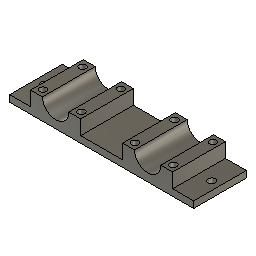
solenoid_railmount v2 (Autodesk Fusion 360 design; units mm, degrees)
Autodesk Fusion 360 part; units mm, degrees
note: some values were not read from the file. Set by a fixed rule: the direction of a hole.
sketch "Sketch1" plane through (0, 0, 0) normal (0, 0, 1) x (1, 0, 0)
  line L0 (0, 0) -> (139.7, 0)
  line L1 (139.7, 0) -> (139.7, 40)
  line L2 (139.7, 40) -> (0, 40)
  line L3 (0, 40) -> (0, 0)
  dimension "d1" = 139.7
  dimension "d2" = 40
  constraint horizontal L0
  constraint vertical L1
  constraint horizontal L2
  constraint vertical L3
  constraint coincident L0.start L3.end
  measures "d1" distance of L0.start L0.end
  measures "d2" distance of L0.start L2.end
extrude "Extrude1" add sketch "Sketch1" along normal blind 5
sketch "Sketch2" plane through (0, 0, 0) normal (0, 0, 1) x (1, 0, 0)
  point P0 (6.35, 20)
  point P1 (133.35, 20)
  constraint horizontal P0 P1
hole "Hole1" at (6.35, 20, 0) at (133.35, 20, 0) direction (0, 0, 1) diameter 5.5 depth 13 tip angle 118 counterbore diameter 9.1 counterbore depth 1
sketch "Sketch7" plane through (0, 0, 5) normal (0, 0, 1) x (-1, 0, 0)
  circle A0 centre (-6.35, -20) radius 2.75
  circle A1 centre (-133.35, -20) radius 2.75
  line L0 (0, -40) -> (0, 0)
  line L1 (0, 0) -> (-139.7, 0)
  line L2 (-139.7, 0) -> (-139.7, -40)
  line L3 (-139.7, -40) -> (0, -40)
  line L4 (-85.775, -40) -> (-123.775, -40)
  line L5 (-123.775, -40) -> (-123.775, 0)
  line L6 (-123.775, 0) -> (-85.775, 0)
  line L7 (-85.775, 0) -> (-85.775, -40)
  line L8 (-85.775, -40) -> (-123.775, 0) construction
  line L9 (-123.775, -40) -> (-85.775, 0) construction
  line L10 (-15.925, -40) -> (-53.925, -40)
  line L11 (-53.925, -40) -> (-53.925, 0)
  line L12 (-53.925, 0) -> (-15.925, 0)
  line L13 (-15.925, 0) -> (-15.925, -40)
  line L14 (-15.925, -40) -> (-53.925, 0) construction
  line L15 (-53.925, -40) -> (-15.925, 0) construction
  point P0 (-104.775, -20)
  point P1 (-34.925, -20)
  point P2 (-104.775, -20)
  point P3 (-34.925, -20)
  dimension "d25" = 38
  dimension "d26" = 40
  dimension "d27" = 38
  dimension "d28" = 40
  constraint horizontal L4
  constraint perpendicular L4 L5
  constraint parallel L4 L6
  constraint parallel L5 L7
  constraint coincident L8 P2
  constraint coincident L9 P2
  constraint coincident P2 P0
  constraint horizontal L10
  constraint perpendicular L10 L11
  constraint parallel L10 L12
  constraint parallel L11 L13
  constraint coincident L14 P3
  constraint coincident L15 P3
  constraint coincident P3 P1
  measures "d25" distance of L5.end L6.end
  measures "d26" distance of L4.end L5.end
  measures "d27" distance of L11.end L12.end
  measures "d28" distance of L10.end L11.end
extrude "Extrude4" add sketch "Sketch7" along normal blind 11 contours L1 L3 L10 L11 L12 L13 | L1 L3 L4 L5 L6 L7
sketch "Sketch8" plane through (0, 40, 0) normal (0, 1, 0) x (-1, 0, 0)
  line L0 (-139.7, 0) -> (0, 0)
  line L1 (0, 0) -> (0, 5)
  line L2 (0, 5) -> (-15.925, 5)
  line L3 (-15.925, 5) -> (-15.925, 16)
  line L4 (-15.925, 16) -> (-53.925, 16)
  line L5 (-53.925, 16) -> (-53.925, 5)
  line L6 (-53.925, 5) -> (-85.775, 5)
  line L7 (-85.775, 5) -> (-85.775, 16)
  line L8 (-85.775, 16) -> (-123.775, 16)
  line L9 (-123.775, 16) -> (-123.775, 5)
  line L10 (-123.775, 5) -> (-139.7, 5)
  line L11 (-139.7, 5) -> (-139.7, 0)
  circle A0 centre (-104.775, 16) radius 10
  circle A1 centre (-34.925, 16) radius 10
  point P0 (-104.775, 16)
  point P1 (-34.925, 16)
  dimension "d31" = 20
  dimension "d32" = 20
  constraint coincident L8 P0
  constraint midpoint L4 P1
  constraint coincident P0 A0.centre
  constraint coincident P1 A1.centre
  measures "d31" diameter of A0
  measures "d32" diameter of A1
extrude "Extrude5" cut sketch "Sketch8" against normal blind 400 contours L8 A0 | L4 A1 picked at (-104.876, 11.6935) picked at (-35.1741, 12.676)
sketch "Sketch9" plane through (0, 0, 16) normal (0, 0, 1) x (-1, 0, 0)
  line L0 (-24.925, 0) -> (-24.925, -40)
  line L1 (-24.925, -40) -> (-15.925, -40)
  line L2 (-15.925, -40) -> (-15.925, 0)
  line L3 (-15.925, 0) -> (-24.925, 0)
  point P0 (-20.375, -5)
  point P1 (-20.375, -35)
  point P2 (-49.475, -5)
  point P3 (-49.475, -35)
  point P4 (-90.225, -35)
  point P5 (-90.225, -5)
  point P6 (-119.325, -35)
  point P7 (-119.325, -5)
  constraint vertical P0 P1
  constraint vertical P2 P3
  constraint vertical P4 P5
  constraint vertical P6 P7
hole "Hole4" at (20.375, 35, 16) at (20.375, 5, 16) at (49.475, 5, 16) at (49.475, 35, 16) at (90.225, 35, 16) at (90.225, 5, 16) at (119.325, 5, 16) at (119.325, 35, 16) direction (0, 0, -1) diameter 5.1 depth 11 tip angle 180
